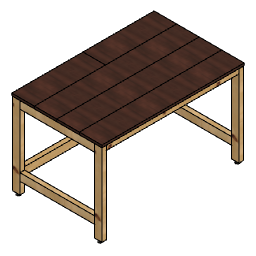
Quick Desk build v12 (Autodesk Fusion 360 design; units mm, degrees)
Autodesk Fusion 360 part; units mm, degrees
note: some values were not read from the file. Chosen so that the rebuilt part matches the saved one: which bodies a step acts on.
sketch "Side" plane through (0, 0, 0) normal (0, 1, 0) x (1, 0, 0)
  line L0 (0, 0) -> (63, 0)
  line L1 (63, 0) -> (63, -690)
  line L2 (63, -690) -> (0, -690)
  line L3 (0, -690) -> (0, 0)
  line L4 (63, -690) -> (691, -690)
  line L5 (691, -690) -> (691, -627)
  line L6 (691, -627) -> (63, -627)
  line L7 (63, -627) -> (63, -690)
  line L8 (691, -690) -> (754, -690)
  line L9 (754, -690) -> (754, 0)
  line L10 (754, 0) -> (691, 0)
  line L11 (691, 0) -> (691, -690)
  line L12 (63, -100) -> (691, -100)
  line L13 (691, -100) -> (691, -163)
  line L14 (691, -163) -> (63, -163)
  line L15 (63, -163) -> (63, -100)
  point P0 (63, -100)
  dimension "d17" = 63
  dimension "d18" = 690
  dimension "d19" = 628
  dimension "d20" = 63
  dimension "d21" = 63
  dimension "d22" = 690
  dimension "d24" = 100
  dimension "d25" = 628
  dimension "d26" = 63
  constraint horizontal L0
  constraint vertical L1
  constraint horizontal L2
  constraint vertical L3
  constraint coincident L0.start L3.end
  constraint horizontal L4
  constraint vertical L5
  constraint horizontal L6
  constraint vertical L7
  constraint horizontal L8
  constraint vertical L9
  constraint horizontal L10
  constraint vertical L11
  constraint coincident L1 P0
  constraint horizontal L12
  constraint vertical L13
  constraint horizontal L14
  constraint vertical L15
  constraint coincident P0 L12.start
  measures "d17" distance of L0.start L0.end
  measures "d18" distance of L0.start L2.end
  measures "d19" distance of L1.end L4.end
  measures "d20" distance of L1.end L6.end
  measures "d21" distance of L4.end L8.end
  measures "d22" distance of L4.end L10.end
  measures "d24" distance of L0.end P0
  measures "d25" distance of P0 L12.end
  measures "d26" distance of P0 L14.end
extrude "Extrude1" add sketch "Side" along normal blind 38 contours L0 L1 L2 L3 L7 L15 | L5 L8 L9 L10 L11 L13 makes body 1 at (21, 0, 460) makes body 2 at (712, 0, 230)
extrude "Extrude2" add sketch "Side" along normal blind 38 separate body contours L1 L11 L12 L13 L14 L15 | L1 L4 L5 L6 L7 L11 makes body 3 at (272.3333, 0, 669) makes body 4 at (272.3333, 0, 121)
pattern_linear "R-Pattern1" count 2 spacing 1156 along (0, 1, 0) of bodies 1 3 2 4 makes body 5 at (21, 1156, 460) makes body 6 at (712, 1156, 230) makes body 7 at (272.3333, 1156, 669) makes body 8 at (272.3333, 1156, 121)
sketch "TopBackBrace" plane through (0, 1156, 0) normal (0, -1, 0) x (1, 0, 0)
  line L0 (63, 0) -> (63, 690)
  line L1 (63, 690) -> (0, 690)
  line L2 (0, 690) -> (0, 0)
  line L3 (0, 0) -> (63, 0)
  line L4 (0, 690) -> (38, 690)
  line L5 (38, 690) -> (38, 627)
  line L6 (38, 627) -> (0, 627)
  line L7 (0, 627) -> (0, 690)
  dimension "d35" = 38
  dimension "d36" = 63
  constraint horizontal L4
  constraint vertical L5
  constraint horizontal L6
  constraint vertical L7
  constraint coincident L1.end L2.start
  measures "d35" distance of L1.end L4.end
  measures "d36" distance of L1.end L6.end
extrude "Extrude3" add sketch "TopBackBrace" along normal blind 1118 separate body contours L1 L2 L4 L5 L6 L7 makes body 9
sketch "BottomBackBrace" plane through (0, 1156, 0) normal (0, -1, 0) x (1, 0, 0)
  line L0 (63, 0) -> (63, 690)
  line L1 (63, 690) -> (0, 690)
  line L2 (0, 690) -> (0, 0)
  line L3 (0, 0) -> (63, 0)
  line L4 (0, 100) -> (38, 100)
  line L5 (38, 100) -> (38, 163)
  line L6 (38, 163) -> (0, 163)
  line L7 (0, 163) -> (0, 100)
  point P0 (0, 100)
  point P1 (63, 100)
  dimension "d39" = 38
  dimension "d40" = 63
  constraint coincident L2 P0
  constraint horizontal P0 P1
  constraint horizontal L4
  constraint vertical L5
  constraint horizontal L6
  constraint vertical L7
  constraint coincident P0 L4.start
  measures "d39" distance of P0 L4.end
  measures "d40" distance of P0 L6.end
extrude "Extrude4" add sketch "BottomBackBrace" along normal blind 1118 separate body contours L2 L4 L5 L6 L7 makes body 10
ref_plane "WorkPlane1" through (31.5, 19, 690) normal (0, 0, 1) x (1, 0, 0)
sketch "TopFrontBrace" plane through (0, 1156, 0) normal (0, -1, 0) x (1, 0, 0)
  line L0 (691, 690) -> (691, 0)
  line L1 (691, 0) -> (754, 0)
  line L2 (754, 0) -> (754, 690)
  line L3 (754, 690) -> (691, 690)
  line L4 (754, 690) -> (691, 690)
  line L5 (691, 690) -> (691, 652)
  line L6 (691, 652) -> (754, 652)
  line L7 (754, 652) -> (754, 690)
  dimension "d50" = 63
  dimension "d51" = 38
  constraint horizontal L4
  constraint vertical L5
  constraint horizontal L6
  constraint vertical L7
  constraint coincident L2.end L3.start
  measures "d50" distance of L2.end L0.start
  measures "d51" distance of L2.end L6.end
extrude "Extrude6" add sketch "TopFrontBrace" along normal blind 1118 separate body contours L0 L2 L3 L4 L5 L6 L7 makes body 11
sketch "Flooring" plane through (0, 0, 0) normal (0, 0, 1) x (1, 0, 0)
  line L0 (0, 0) -> (1200, 0)
  line L1 (1200, 0) -> (1200, 190)
  line L2 (1200, 190) -> (0, 190)
  line L3 (0, 190) -> (0, 0)
  line L4 (1200, 0) -> (1900, 0)
  line L5 (1900, 0) -> (1900, 190)
  line L6 (1900, 190) -> (1200, 190)
  line L7 (1200, 190) -> (1200, 0)
  line L8 (0, 190) -> (1200, 190)
  line L9 (1200, 190) -> (1200, 380)
  line L10 (1200, 380) -> (0, 380)
  line L11 (0, 380) -> (0, 190)
  line L12 (1200, 190) -> (1900, 190)
  line L13 (1900, 190) -> (1900, 380)
  line L14 (1900, 380) -> (1200, 380)
  line L15 (1200, 380) -> (1200, 190)
  line L16 (0, 380) -> (1200, 380)
  line L17 (1200, 380) -> (1200, 570)
  line L18 (1200, 570) -> (0, 570)
  line L19 (0, 570) -> (0, 380)
  line L20 (1200, 380) -> (1500, 380)
  line L21 (1500, 380) -> (1500, 570)
  line L22 (1500, 570) -> (1200, 570)
  line L23 (1200, 570) -> (1200, 380)
  line L24 (600, 570) -> (-100, 570)
  line L25 (-100, 570) -> (-100, 760)
  line L26 (-100, 760) -> (600, 760)
  line L27 (600, 760) -> (600, 570)
  line L28 (600, 570) -> (1300, 570)
  line L29 (1300, 570) -> (1300, 760)
  line L30 (1300, 760) -> (600, 760)
  line L31 (600, 760) -> (600, 570)
  line L32 (0, 570) -> (0, 760)
  line L33 (1200, 570) -> (1200, 760)
  point P0 (600, 570)
  dimension "d54" = 1200
  dimension "d55" = 190
  dimension "d56" = 700
  dimension "d57" = 190
  dimension "d58" = 190
  dimension "d59" = 1200
  dimension "d60" = 190
  dimension "d61" = 300
  dimension "d62" = 700
  dimension "d63" = 190
  dimension "d64" = 700
  constraint horizontal L0
  constraint vertical L1
  constraint horizontal L2
  constraint vertical L3
  constraint coincident L0.start L3.end
  constraint horizontal L4
  constraint vertical L5
  constraint horizontal L6
  constraint vertical L7
  constraint horizontal L8
  constraint vertical L9
  constraint horizontal L10
  constraint vertical L11
  constraint horizontal L12
  constraint vertical L13
  constraint horizontal L14
  constraint vertical L15
  constraint horizontal L16
  constraint vertical L17
  constraint horizontal L18
  constraint vertical L19
  constraint horizontal L20
  constraint vertical L21
  constraint horizontal L22
  constraint vertical L23
  constraint midpoint L18 P0
  constraint horizontal L24
  constraint vertical L25
  constraint horizontal L26
  constraint vertical L27
  constraint coincident P0 L24.start
  constraint horizontal L28
  constraint vertical L29
  constraint horizontal L30
  constraint vertical L31
  constraint coincident L26 L32.end
  constraint perpendicular L26 L32
  constraint coincident L30 L33.end
  constraint perpendicular L30 L33
  measures "d54" distance of L0.start L0.end
  measures "d55" distance of L0.start L2.end
  measures "d56" distance of L0.end L4.end
  measures "d57" distance of L2.end L10.end
  measures "d58" distance of L1.end L9.end
  measures "d59" distance of L10.end L9.end
  measures "d60" distance of L10.end L18.end
  measures "d61" distance of L9.end L20.end
  measures "d62" distance of P0 L24.end
  measures "d63" distance of P0 L26.end
  measures "d64" distance of P0 L28.end
extrude "Extrude7" add sketch "Flooring" along normal blind 20 separate body contours L0 L1 L2 L3 L7 L8 makes body 12
extrude "Extrude8" add sketch "Flooring" along normal blind 20 separate body contours L2 L8 L9 L10 L11 L15 L16 makes body 13
extrude "Extrude9" add sketch "Flooring" along normal blind 20 separate body contours L10 L16 L17 L18 L19 L23 L24 L28 makes body 14
extrude "Extrude10" add sketch "Flooring" along normal blind 20 separate body contours L18 L24 L26 L27 L31 L32 makes body 15
extrude "Extrude11" add sketch "Flooring" along normal blind 20 separate body contours L18 L27 L28 L30 L31 L33 makes body 16
move_body "Move4" bodies 12 13 14 15 16 to x (0, 1, 0) y (-1, 0, 0) z (0, 0, 1) at (0, 0, 0)
move_body "Move5" bodies 12 13 14 15 16 to x (1, 0, 0) y (0, 1, 0) z (0, 0, 1) at (754, 0, 690)
move_body "Move6" bodies 1 4 14 7 8 3 5 9 2 16 11 10 6 13 15 12 to x (1, 0, 0) y (0, 1, 0) z (0, 0, 1) at (0, 0, 20)
sketch "LevelFeet" plane through (0, 0, 20) normal (0, 0, -1) x (1, 0, 0)
  line L0 (63, 0) -> (0, 0)
  line L1 (0, 0) -> (0, -38)
  line L2 (0, -38) -> (63, -38)
  line L3 (63, -38) -> (63, 0)
  circle A0 centre (31.5, -19) radius 16
  circle A1 centre (722.5, -19) radius 16
  circle A2 centre (31.5, -1175) radius 16
  circle A3 centre (722.5, -1175) radius 16
  point P0 (31.5, -19)
  dimension "d81" = 32
  dimension "d82" = 32
  dimension "d83" = 691
  dimension "d84" = 32
  dimension "d85" = 1156
  dimension "d86" = 32
  dimension "d87" = 691
  constraint coincident P0 A0.centre
  measures "d81" diameter of A0
  measures "d82" diameter of A1
  measures "d83" distance of P0 A1.centre
  measures "d84" diameter of A2
  measures "d85" distance of P0 A2.centre
  measures "d86" diameter of A3
  measures "d87" distance of A2.centre A3.centre
extrude "Extrude12" add sketch "LevelFeet" along normal blind 20 separate body contours A0 | A1 | A2 | A3 makes body 17 at (711.3282, 7.5461, 6.6667) makes body 18 at (706.9948, 1171.0519, 6.6667) makes body 19 at (47.4801, 19.7975, 6.6667) makes body 20 at (15.8172, 1171.8297, 13.3333)
equation "CLSWidth = 63 mm"
equation "CLSThickness = 38 mm"
equation "IdealHeight = 730 mm"
equation "DeskTopThickness = 20 mm"
equation "DeskTopPlankWidth = 190 mm"
equation "LevelFeetHeight = 20 mm"
equation "LevelFeetDia = 32 mm"
equation "DeskWidth = 1200 mm"
equation "DeskDepth = DeskTopPlankWidth * 4"
equation "BackBraceLength = DeskWidth - ( CLSThickness * 2 ) - TrimFloorGroove"
equation "SideBraceLength = DeskDepth - ( CLSWidth * 2 ) - TrimFloorGroove"
equation "LegHeight = IdealHeight - DeskTopThickness - LevelFeetHeight"
equation "d17 = CLSWidth"
equation "d18 = LegHeight"
equation "d19 = SideBraceLength"
equation "d20 = CLSWidth"
equation "d21 = CLSWidth"
equation "d22 = LegHeight"
equation "BottomBraceStartFromBottom = 100 mm"
equation "d24 = BottomBraceStartFromBottom"
equation "d25 = SideBraceLength"
equation "d26 = CLSWidth"
equation "d27 = CLSThickness"
equation "d29 = CLSThickness"
equation "d33 = BackBraceLength + CLSThickness"
equation "d34 = DeskWidth"
equation "d35 = CLSThickness"
equation "d36 = CLSWidth"
equation "d37 = BackBraceLength"
equation "d39 = CLSThickness"
equation "d40 = CLSWidth"
equation "d41 = BackBraceLength"
equation "d50 = CLSWidth"
equation "d51 = CLSThickness"
equation "d52 = BackBraceLength"
equation "d56 = 1900 mm - 1200 mm"
equation "d61 = 1500 mm - 1200 mm"
equation "d65 = DeskTopThickness"
equation "d67 = DeskTopThickness"
equation "d69 = DeskTopThickness"
equation "d71 = DeskTopThickness"
equation "d73 = DeskTopThickness"
equation "TrimFloorGroove = 6 mm"
equation "d80 = LevelFeetHeight"
equation "d81 = LevelFeetDia"
equation "d82 = LevelFeetDia"
equation "d83 = SideBraceLength + CLSWidth"
equation "d84 = LevelFeetDia"
equation "d85 = BackBraceLength + CLSThickness"
equation "d86 = LevelFeetDia"
equation "d87 = SideBraceLength + CLSWidth"
equation "d88 = LevelFeetHeight"
named bodies: "LhsBackLeg", "LhsFrontLeg", "LhsSideBraceTop", "LhsSideBraceBottom", "RhsBackLeg", "RhsFrontLeg", "RhsSideBraceTop", "RhsSideBraceBottom", "BackBraceTop", "BackBraceBottom", "TopFrontBrace"
